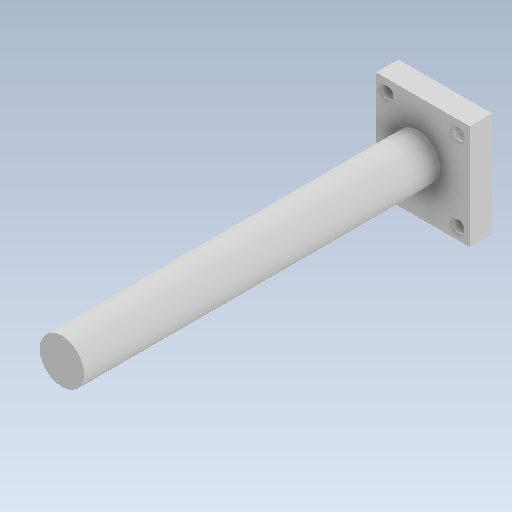
# Autodesk Inventor part: Part8
Saved by Autodesk Inventor 2020.2 (Build 242310000, 310)
## iProperties
Created: 2022-11-03
Part Number: Part8
Material: 一般
Document SubType Name: Modeling
Designer: Administrator
Density: 1 g/cm^3
Appearance: 既定
Author: Administrator
Autodesk Inventor part; units mm, degrees
ref_plane "YZ Plane" through (0, 0, 0) normal (1, 0, 0) x (0, 1, 0)
ref_plane "XZ Plane" through (0, 0, 0) normal (0, 1, 0) x (-1, 0, 0)
ref_plane "XY Plane" through (0, 0, 0) normal (0, 0, 1) x (1, 0, 0)
sketch "スケッチ1" plane through (0, 0, 0) normal (0, 0, 1) x (1, 0, 0)
  circle A0 centre (37, 36) radius 2.75 projected
  line L0 (42, 30.5) -> (42, 41.5) projected
  line L1 (28, 41.5) -> (42, 41.5) projected
  line L2 (28, 30.5) -> (28, 41.5) projected
  line L3 (42, 30.5) -> (28, 30.5) projected
  circle A1 centre (5, 36) radius 2.75 projected
  line L4 (14, 30.5) -> (14, 41.5) projected
  line L5 (0, 41.5) -> (14, 41.5) projected
  line L6 (0, 30.5) -> (0, 41.5) projected
  line L7 (14, 30.5) -> (0, 30.5) projected
  circle A2 centre (37, 0) radius 2.75 projected
  line L8 (42, -5.5) -> (42, 5.5) projected
  line L9 (28, 5.5) -> (42, 5.5) projected
  line L10 (28, -5.5) -> (28, 5.5) projected
  line L11 (42, -5.5) -> (28, -5.5) projected
  circle A3 centre (5, 0) radius 2.75 projected
  line L12 (14, -5.5) -> (14, 5.5) projected
  line L13 (0, 5.5) -> (14, 5.5) projected
  line L14 (0, -5.5) -> (0, 5.5) projected
  line L15 (14, -5.5) -> (0, -5.5) projected
  line L16 (0, -5.5) -> (42, -5.5)
  line L17 (42, -5.5) -> (42, 41.5)
  line L18 (42, 41.5) -> (0, 41.5)
  line L19 (0, 41.5) -> (0, -5.5)
  point P0 (0, 0)
  constraints: 8 end point, 2 parallel, 1 horizontal, 1 perpendicular
extrude "押し出し1" add sketch "スケッチ1" along normal blind 10
sketch "スケッチ2" plane through (0, 0, 10) normal (0, 0, 1) x (1, 0, 0)
  circle A0 centre (18.766, 18.4051) radius 10
  point P0 (0, 0)
  dimension "d2" = 20
  constraints: 1 centre point
  measures "d2" diameter of A0
extrude "押し出し2" add sketch "スケッチ2" along normal blind 160
